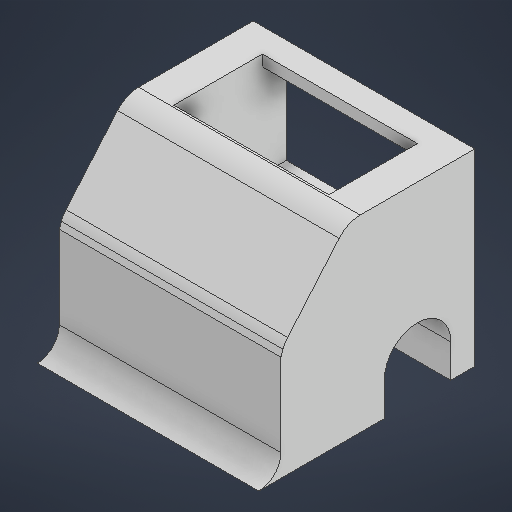
# Autodesk Inventor part: Mini-sumô rascunho
Saved by Autodesk Inventor 2026.1 (Build 301233000, 233)
## iProperties
Created: 2025-10-23
Part Number: Mini-sumô rascunho
Material: Genérico
Document SubType Name: Modeling
Designer: panto
Density: 1 g/cm^3
Appearance: Padrão
Author: panto
Autodesk Inventor part; units mm, degrees
ref_plane "YZ Plane" through (0, 0, 0) normal (1, 0, 0) x (0, 1, 0)
ref_plane "XZ Plane" through (0, 0, 0) normal (0, 1, 0) x (-1, 0, 0)
ref_plane "XY Plane" through (0, 0, 0) normal (0, 0, 1) x (1, 0, 0)
sketch "Esboço1" plane through (0, 0, 0) normal (0, 1, 0) x (-1, 0, 0)
  line L0 (0, 0) -> (-100, 0)
  line L1 (-100, 0) -> (-100, -100)
  line L2 (-100, -100) -> (0, -100)
  line L3 (0, -100) -> (0, 0)
  dimension "d0" = 100
  dimension "d1" = 100
  constraints: 8 end point, 2 parallel, 1 horizontal, 1 perpendicular
  measures "d0" distance of L2.end L1.end
  measures "d1" distance of L1.end L0.end
extrude "Extrusão1" add sketch "Esboço1" along normal blind 85
sketch "Esboço2" plane through (100, 0, 0) normal (1, 0, 0) x (0, 0, -1)
  line L0 (0, 0) -> (100, 0) projected
  line L1 (0, 0) -> (2.5, 0)
  line L2 (12.5, 10) -> (12.5, 45.3759)
  line L3 (0, 85) -> (100, 85) projected
  line L4 (12.5, 50) -> (13.3867, 50)
  line L5 (42.5, 85) -> (12.5, 85)
  line L6 (12.5, 85) -> (12.5, 50)
  line L7 (15.5093, 53.5108) -> (38.7585, 80.6349)
  arc A0 (2.5, 0) -> (12.5, 10) centre (2.5, 10) ccw
  line L8 (2.5, 0) -> (100, 0)
  line L9 (48.2492, 85) -> (100, 85)
  line L10 (100, 85) -> (100, 0)
  arc A1 (15.5093, 53.5108) -> (12.5, 45.3759) centre (25, 45.3759) ccw
  line L11 (12.5, 85) -> (42.5, 85)
  line L12 (12.5, 85) -> (0, 85)
  arc A2 (48.2492, 85) -> (38.7585, 80.6349) centre (48.2492, 72.5) ccw
  circle A3 centre (74.1246, 15) radius 15
  line L13 (0, 85) -> (0, 0)
  line L14 (0, 0) -> (2.5, 0)
  line L15 (59.1246, 15) -> (59.1246, 0)
  line L16 (89.1246, 15) -> (89.1246, 0)
  line L17 (12.5, 50) -> (12.5, 45.3759)
  line L18 (12.5, 85) -> (48.2492, 85)
  point P0 (12.5, 0)
  dimension "d4" = 12.5
  dimension "d7" = 10
  dimension "d8" = 12.5
  dimension "d9" = 12.5
  dimension "d11" = 30
  constraints: 34 end point, 11 tangent, 10 point on line, 9 point on circle, 5 collinear, 5 perpendicular, 4 centre point, 1 horizontal, 1 parallel, 1 vertical
  measures "d4" distance of L0.start point (12.5, 0)
  measures "d7" radius of A0
  measures "d8" radius of A1
  measures "d9" radius of A2
  measures "d11" diameter of A3
extrude "Extrusão2" cut sketch "Esboço2" against normal blind 100 contours L13 L3 L6 L17 L2 A0 L0 | L3 A2 L7 A1 L4 L6
extrude "Extrusão3" cut sketch "Esboço2" against normal blind 30 contours L15 A3 L0 | A3 L16 L0 | A3
sketch "Esboço3" plane through (0, 0, -100) normal (-1, 0, 0) x (0, 0, 1)
  line L0 (86.6133, 50) -> (87.5, 50)
  arc A0 (86.6133, 50) -> (84.4907, 53.5108) centre (75, 45.3759) ccw projected
  line L1 (86.6133, 50) -> (87.5, 47.3246)
  line L2 (87.5, 50) -> (87.5, 10) projected
  line L3 (86.6133, 50) -> (87.5, 50)
  line L4 (87.5, 50) -> (87.5, 47.3246)
  arc A1 (40.8754, 15) -> (10.8754, 15) centre (25.8754, 15) ccw projected
  circle A2 centre (25.8754, 15) radius 15
  line L5 (10.8754, 15) -> (10.8754, 0) projected
  line L6 (10.8754, 15) -> (10.8754, 0)
  line L7 (97.5, 0) -> (40.8754, 0) projected
  line L8 (40.8754, 15) -> (40.8754, 0)
  line L9 (10.8754, 0) -> (40.8754, 0)
  point P0 (100, 0)
  constraints: 14 end point, 3 collinear, 2 perpendicular, 1 centre point, 1 coincident, 1 horizontal, 1 point on line, 1 tangent
extrude "Extrusão4" cut sketch "Esboço3" against normal blind 30 contours A2 A1 | L8 L9 A2 | A2 L9 L5
extrude "Extrusão5" cut sketch "Esboço3" against normal blind 100 contours L0 L2 L1
sketch "Esboço4" plane through (100, 0, -100) normal (0, 0, -1) x (-1, 0, 0)
  line L0 (15, 35) -> (85, 35)
  line L1 (15, 35) -> (15, 80)
  line L2 (0, 53.5108) -> (100, 53.5108) projected
  line L3 (15, 35) -> (60, 35) construction
  line L4 (15, 80) -> (85, 80)
  line L5 (85, 80) -> (85, 35)
  line L6 (70, 30) -> (70, 15) projected
  line L7 (15, 35) -> (15, 38)
  line L8 (15, 38) -> (85, 38)
  line L9 (0, 0) -> (0, 85) projected
  line L10 (0, 35) -> (50, 35)
  line L11 (37.5, 35) -> (35, 35)
  line L12 (35, 35) -> (35, 22.5)
  line L13 (35, 22.5) -> (65, 22.5)
  line L14 (65, 22.5) -> (65, 35)
  line L15 (35, 22.5) -> (35, 24.5)
  line L16 (35, 24.5) -> (65, 24.5)
  dimension "d26" = 70
  dimension "d27" = 45
  dimension "d31" = 3
  dimension "d34" = 30
  dimension "d35" = 2
  constraints: 28 end point, 8 point on line, 7 perpendicular, 4 horizontal, 1 midpoint
  measures "d26" distance of L0.start L0.end
  measures "d27" distance of L0.start L1.end
  measures "d31" distance of L0.start L7.end
  measures "d34" distance of L12.end L13.end
  measures "d35" distance of L12.end L15.end
extrude "Extrusão6" cut sketch "Esboço4" against normal blind 60 contours L0 L14 L16 L12 | L1 L2 L5 L8 | L1 L4 L5 L2
sketch "Esboço5" plane through (0, 85, 0) normal (0, 1, 0) x (1, 0, 0)
  line L0 (100, 89.1246) -> (70, 89.1246) projected
  line L1 (85, 89.1246) -> (85, 49.1246)
  line L2 (85, 100) -> (85, 40) projected
  line L3 (85, 49.1246) -> (15, 49.1246)
  line L4 (15, 100) -> (15, 40) projected
  line L5 (15, 49.1246) -> (15, 89.1246)
  line L6 (15, 89.1246) -> (85, 89.1246)
  point P0 (0, 0)
  dimension "d38" = 40
  constraints: 8 end point, 2 perpendicular, 2 point on line, 1 midpoint, 1 vertical
  measures "d38" distance of L1.start L1.end
extrude "Extrusão7" cut sketch "Esboço5" against normal blind 30
